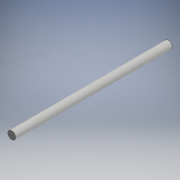
# Autodesk Inventor part: reifen_achse
Saved by Autodesk Inventor 2018 (Build 220112000, 112)
## iProperties
Created: 2020-03-17
Part Number: reifen_achse
Material: Generisch
Document SubType Name: Blech
Designer: wepet
Density: 1 g/cm^3
Sheet Metal Rule: Standard_mm
Appearance: Vorgabe
Author: wepet
Autodesk Inventor part; units mm, degrees
ref_plane "YZ Plane" through (0, 0, 0) normal (1, 0, 0) x (0, 1, 0)
ref_plane "XZ Plane" through (0, 0, 0) normal (0, 1, 0) x (-1, 0, 0)
ref_plane "XY Plane" through (0, 0, 0) normal (0, 0, 1) x (1, 0, 0)
sketch "Skizze1" plane through (0, 0, 0) normal (0, 1, 0) x (-1, 0, 0)
  circle A0 centre (0, 0) radius 4
  dimension "d0" = 8
  constraints: 1 centre point, 1 coincident
  measures "d0" diameter of A0
extrude "reifen_achse" add sketch "Skizze1" along normal blind 160
equation "\"Biegeradius\" = Stärke"
equation "\"BreiteBiegungsfreistellung\" = Stärke"
equation "\"TiefeBiegungsfreistellung\" = 0.5 * Stärke"
equation "\"GrößeEckenfreistellung\" = 4 * Stärke"
equation "\"MinimalRest\" = 2 * Stärke"
equation "\"Übergangsradius\" = Biegeradius"
equation "\"JacobiRadiusGröße\" = Biegeradius"
equation "\"Abstandsgröße\" = Stärke"
equation "\"Stärke\" = 0.5"
